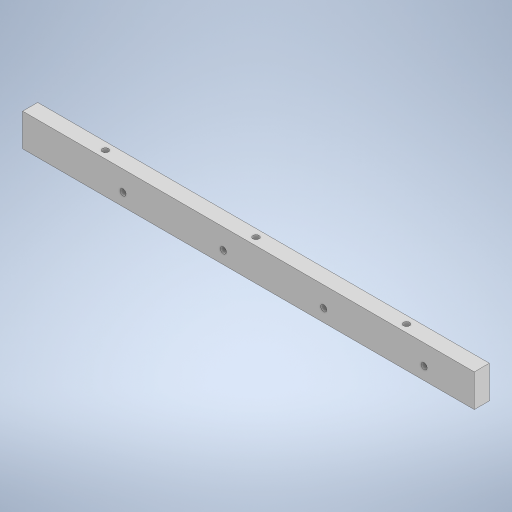
# Autodesk Inventor part: slider
Saved by Autodesk Inventor 2023 (Build 270158000, 158)
## iProperties
Created: 2022-12-04
Part Number: slider
Material: 一般
Document SubType Name: Modeling
Designer: RiSA
Density: 1 g/cm^3
Appearance: 既定
Author: RiSA
Autodesk Inventor part; units mm, degrees
ref_plane "YZ Plane" through (0, 0, 0) normal (1, 0, 0) x (0, 1, 0)
ref_plane "XZ Plane" through (0, 0, 0) normal (0, 1, 0) x (-1, 0, 0)
ref_plane "XY Plane" through (0, 0, 0) normal (0, 0, 1) x (1, 0, 0)
sketch "スケッチ2" plane through (0, 0, 0) normal (0, 1, 0) x (-1, 0, 0)
  line L0 (-90, -3) -> (90, -3)
  line L1 (90, -3) -> (90, 3)
  line L2 (90, 3) -> (-90, 3)
  line L3 (-90, 3) -> (-90, -3)
  line L4 (-90, -3) -> (90, 3) construction
  line L5 (90, -3) -> (-90, 3) construction
  point P0 (0, 0)
  dimension "d1" = 180
  dimension "d2" = 6
  constraints: 12 end point, 2 midpoint, 2 parallel, 1 horizontal, 1 perpendicular
  measures "d1" distance of L2.end L1.end
  measures "d2" distance of L1.end L0.end
extrude "押し出し1" add sketch "スケッチ2" along normal blind 13
sketch "スケッチ3" plane through (-90, 0, 3) normal (0, 0, 1) x (1, 0, 0)
  line L0 (0, 0) -> (180, 0) projected
  line L1 (180, 0) -> (180, 13) projected
  point P0 (90, 0)
  point P1 (160, 5)
  point P2 (120, 5)
  point P3 (80, 5)
  point P4 (40, 5)
  dimension "d5" = 5
  dimension "d6" = 20
  dimension "d7" = 40
  dimension "d8" = 40
  dimension "d16" = 40
  dimension "d17" = 5
  measures "d5" distance from line of L0 point (160, 5)
  measures "d6" distance from line of L1 point (160, 5)
  measures "d7" distance of point (160, 5) point (120, 5)
  measures "d8" distance of point (120, 5) point (80, 5)
  measures "d16" distance of point (80, 5) point (40, 5)
  measures "d17" distance from line of L0 point (80, 5)
hole "穴1" at (70, 5, 3) at (30, 5, 3) at (-10, 5, 3) at (-50, 5, 3) direction (0, 0, -1) diameter 2.5 end through all
sketch "スケッチ4" plane through (0, 0, 0) normal (0, -1, 0) x (1, 0, 0)
  line L0 (90, 3) -> (90, -3) projected
  point P0 (0, 0)
  point P1 (60, 0)
  point P2 (0, 0)
  point P3 (-60, 0)
  dimension "d18" = 30
  dimension "d19" = 60
  dimension "d20" = 60
  measures "d18" distance from line of point (60, 0) L0
  measures "d19" distance of point (60, 0) point (0, 0)
  measures "d20" distance of point (0, 0) point (-60, 0)
hole "穴2" at (60, 0, 0) at (0, 0, 0) at (-60, 0, 0) direction (0, 1, 0) diameter 2.5 end through all
